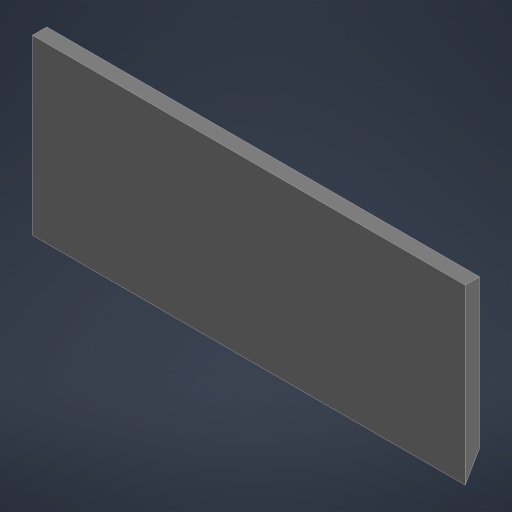
# Autodesk Inventor part: pług_część1
Saved by Autodesk Inventor 2023.4 (Build 274418000, 418)
## iProperties
Created: 2025-10-31
Part Number: pług_część1
Material: Stal
Document SubType Name: Modeling
Designer: Jakub Borsukiewicz
Density: 7.85 g/cm^3
Appearance: Szara
Author: Jakub Borsukiewicz
Autodesk Inventor part; units mm, degrees
ref_plane "YZ Plane" through (0, 0, 0) normal (1, 0, 0) x (0, 1, 0)
ref_plane "XZ Plane" through (0, 0, 0) normal (0, 1, 0) x (-1, 0, 0)
ref_plane "XY Plane" through (0, 0, 0) normal (0, 0, 1) x (1, 0, 0)
sketch "Szkic1" plane through (0, 0, 0) normal (0, 0, 1) x (1, 0, 0)
  line L0 (0, -25.2) -> (0, 25.2) projected
  line L1 (-63, 0) -> (63, 0) projected
  line L2 (-45, -18) -> (45, -18)
  line L3 (45, -18) -> (45, 18)
  line L4 (45, 18) -> (-45, 18)
  line L5 (-45, 18) -> (-45, -18)
  line L6 (-45, -18) -> (45, 18) construction
  line L7 (45, -18) -> (-45, 18) construction
  point P0 (0, 0)
  dimension "d0" = 36
  dimension "d1" = 90
  constraints: 12 end point, 2 midpoint, 2 parallel, 1 horizontal, 1 perpendicular
  measures "d0" distance of L2.end L3.end
  measures "d1" distance of L3.end L4.end
extrude "Wyciągnięcie proste1" add sketch "Szkic1" along normal blind 3
sketch "Szkic3" plane through (45, -18, 0) normal (1, 0, 0) x (0, 0, -1)
  line L0 (-3, 0) -> (-3, 36) projected
  line L1 (0, 0) -> (0, 36) projected
  line L2 (0, 0) -> (0, 36) projected
  line L3 (0, 36) -> (-3, 36) projected
  line L4 (-3, 0) -> (-3, 36) projected
  line L5 (0, 0) -> (-3, 0) projected
  line L6 (-3, 0) -> (0, 5.1962)
  point P0 (0, 18)
  point P1 (0, 5.1962)
  dimension "d10" = 30
  constraints: 2 end point, 1 point on line
  measures "d10" angle of L1 L6
extrude "Wyciągnięcie proste3" cut sketch "Szkic3" against normal blind 100 contours L6 L1 L5
